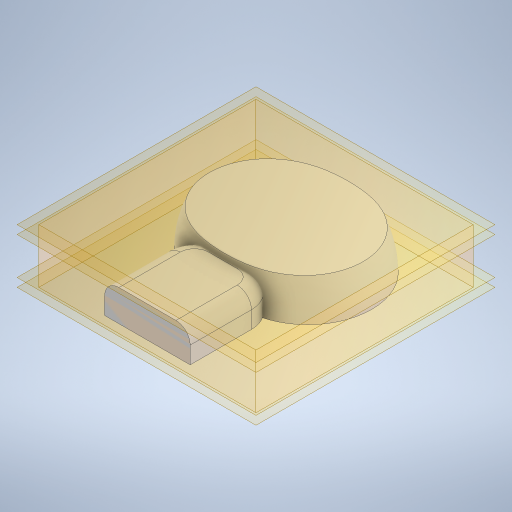
# Autodesk Inventor part: MOLDE
Saved by Autodesk Inventor 2023.2 (Build 272271030, 271C)
## iProperties
Created: 2023-08-26
Part Number: MOLDE
Material: Generic
Document SubType Name: Modeling
Designer: Cris Pat
Density: 1 g/cm^3
Appearance: Default
Author: Cris Pat
Autodesk Inventor part; units mm, degrees
ref_plane "YZ Plane" through (0, 0, 0) normal (1, 0, 0) x (0, 1, 0)
ref_plane "XZ Plane" through (0, 0, 0) normal (0, 1, 0) x (-1, 0, 0)
sketch "Sketch1" plane through (0, 0, 0) normal (0, 0, 1) x (1, 0, 0)
  line L0 (0, 76.2) -> (76.2, 76.2)
  line L1 (76.2, 76.2) -> (76.2, 0)
  line L2 (76.2, 0) -> (0, 0)
  line L3 (0, 0) -> (0, 76.2)
  dimension "d0" = 76.2
  dimension "d1" = 76.2
  constraints: 8 end point, 2 parallel, 1 coincident, 1 horizontal, 1 perpendicular
  measures "d0" distance between parallel lines of L1 L3
  measures "d1" distance between parallel lines of L2 L0
surface extrude "STOCK_LIMITE_PERIMETRAL" sketch "Sketch1" against normal blind 19.05 shown yes curves L3 L0 L1 L2
ref_plane "STOCK_LIMITE_INFERIOR" through (0, 0, -19.05) normal (0, 0, 1) x (1, 0, 0)
ref_plane "PIEZA_LIMITE_SUPERIOR" through (0, 0, -3) normal (0, 0, 1) x (1, 0, 0)
ref_plane "PIEZA_LIMITE_INFERIOR" through (0, 0, -16.05) normal (0, 0, 1) x (1, 0, 0)
sketch "Sketch2" plane through (0, 0, -16.05) normal (0, 0, 1) x (1, 0, 0)
  line L0 (0, 76.2) -> (76.2, 76.2) construction
  line L1 (76.2, 0) -> (0, 0) construction
  line L2 (0, 0) -> (0, 76.2) construction
  line L3 (76.2, 76.2) -> (76.2, 0) construction
  line L4 (6.6, 71.2) -> (69.6, 71.2)
  line L5 (69.6, 71.2) -> (69.6, 26.2)
  line L6 (69.6, 26.2) -> (6.6, 26.2)
  line L7 (6.6, 26.2) -> (6.6, 71.2)
  line L8 (0, 76.2) -> (76.2, 76.2) construction
  point P0 (38.1, 71.2)
  point P1 (38.1, 76.2)
  point P2 (38.1, 76.2)
  dimension "d7" = 45
  dimension "d8" = 63
  dimension "d9" = 5
  constraints: 8 end point, 3 midpoint, 2 parallel, 1 horizontal, 1 perpendicular, 1 vertical alignment
  measures "d7" distance between parallel lines of L6 L4
  measures "d8" distance between parallel lines of L5 L7
  measures "d9" distance of point (38.1, 71.2) point (38.1, 76.2)
extrude "Extrusion1" add sketch "Sketch2" along normal up to surface (13.05 mm away)
fillet "Fillet1" [suppressed]
sketch "Sketch5" plane through (0, 0, -16.05) normal (0, 0, 1) x (1, 0, 0)
  line L0 (6.6, 26.2) -> (6.6, 71.2) construction
  line L1 (69.6, 26.2) -> (6.6, 26.2) construction
  line L2 (69.6, 71.2) -> (69.6, 26.2) construction
  line L3 (6.6, 71.2) -> (69.6, 71.2) construction
  line L4 (38.1, 71.2) -> (38.1, 26.2)
  arc A0 (45.6, 26.2) -> (45.6, 71.2) centre (45.6, 48.7) ccw
  line L5 (45.6, 71.2) -> (38.1, 71.2)
  line L6 (45.6, 26.2) -> (38.1, 26.2)
  point P0 (0, 0)
  point P1 (38.1, 48.7)
  point P2 (68.1, 48.7)
  dimension "d21" = 30
  constraints: 6 end point, 3 midpoint, 3 point on circle, 2 collinear, 2 point on line, 2 tangent, 1 centre point, 1 coincident
  measures "d21" distance of point (38.1, 48.7) point (68.1, 48.7)
revolve "Revolution3" cut sketch "Sketch5" angle 180 about axis through (38.1, 71.2, -16.05) along (0, -1, 0) keep common part
sketch "Sketch6" plane through (0, 0, -16.05) normal (0, 0, 1) x (1, 0, 0)
  arc A0 (30.6, 71.2) -> (30.6, 26.2) centre (30.6, 48.7) ccw construction
  line L0 (45.6, 71.2) -> (30.6, 71.2) construction
  arc A1 (45.6, 26.2) -> (45.6, 71.2) centre (45.6, 48.7) ccw construction
  line L1 (0, 76.2) -> (76.2, 76.2) construction
  line L2 (76.2, 0) -> (0, 0) construction
  line L3 (23.1, 31.5) -> (53.1, 31.5)
  line L4 (53.1, 31.5) -> (53.1, 0)
  line L5 (53.1, 0) -> (23.1, 0)
  line L6 (23.1, 0) -> (23.1, 31.5)
  point P0 (38.1, 31.5)
  point P1 (38.1, 0)
  dimension "d23" = 30
  dimension "d24" = 31.5
  dimension "d25" = 0
  constraints: 8 end point, 2 midpoint, 2 parallel, 1 horizontal, 1 perpendicular, 1 vertical alignment, 1 other
  measures "d23" distance between parallel lines of L4 L6
  measures "d24" distance between parallel lines of L5 L3
  measures "d25" distance between parallel lines of L2 L5
extrude "Extrusion2" add sketch "Sketch6" along normal blind 11 separate body
fillet "Fillet2" radius 10 2 edges at (23.1, 31.5, -10.55) (53.1, 31.5, -10.55)
fillet "Fillet3" radius 5 5 edges at (26.0289, 28.5711, -5.05) (38.1, 31.5, -5.05) (50.1711, 28.5711, -5.05) (53.1, 10.75, -5.05) (23.1, 10.75, -5.05)
equation "\"d8\" = 1.4 * d7"
equation "\"d24\" = 1.05 * d23"
body "Solid1"
body "Srf1"
body "Solid2"
